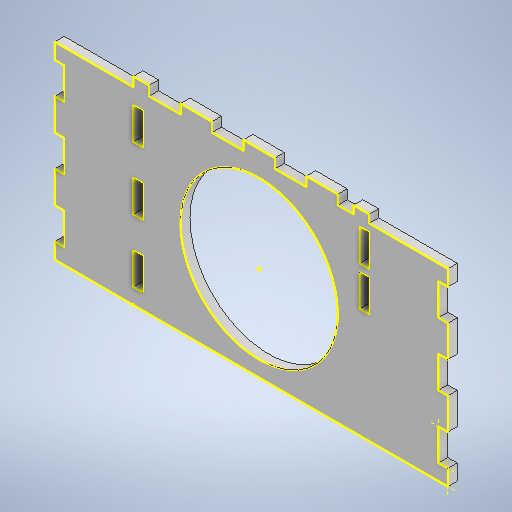
# Autodesk Inventor part: Archimedes Screw Border1
Saved by Autodesk Inventor 2025.3 (Build 293356000, 356)
## iProperties
Created: 2026-03-14
Part Number: Archimedes Screw Border1
Material: Generic
Document SubType Name: Modeling
Designer: ziada
Density: 1 g/cm^3
Appearance: Default
Author: ziada
Autodesk Inventor part; units mm, degrees
ref_plane "YZ Plane" through (0, 0, 0) normal (1, 0, 0) x (0, 1, 0)
ref_plane "XZ Plane" through (0, 0, 0) normal (0, 1, 0) x (-1, 0, 0)
ref_plane "XY Plane" through (0, 0, 0) normal (0, 0, 1) x (1, 0, 0)
sketch "Sketch1" plane through (0, 0, 0) normal (0, 0, 1) x (1, 0, 0)
  line L0 (0, 0) -> (0, 120)
  circle A0 centre (80, 60) radius 50
  line L1 (0, 0) -> (150, 0)
  line L2 (150, 120) -> (0, 120)
  line L3 (0, 120) -> (0, 110)
  line L4 (0, 110) -> (6, 110)
  line L5 (6, 110) -> (6, 90)
  line L6 (6, 90) -> (0, 90)
  line L7 (0, 90) -> (0, 70)
  line L8 (0, 70) -> (6, 70)
  line L9 (6, 70) -> (6, 50)
  line L10 (6, 50) -> (0, 50)
  line L11 (0, 50) -> (0, 30)
  line L12 (0, 30) -> (6, 30)
  line L13 (6, 30) -> (6, 10)
  line L14 (6, 10) -> (0, 10)
  line L15 (0, 120) -> (-50, 120)
  line L16 (-50, 120) -> (-50, 110)
  line L17 (-50, 110) -> (-44, 110)
  line L18 (-44, 110) -> (-44, 90)
  line L19 (-44, 90) -> (-50, 90)
  line L20 (-50, 90) -> (-50, 70)
  line L21 (-50, 70) -> (-44, 70)
  line L22 (-44, 70) -> (-44, 50)
  line L23 (-44, 50) -> (-50, 50)
  line L24 (-50, 50) -> (-50, 30)
  line L25 (-50, 30) -> (-44, 30)
  line L26 (-44, 30) -> (-44, 10)
  line L27 (-44, 10) -> (-50, 10)
  line L28 (-50, 10) -> (-50, 0)
  line L29 (-50, 0) -> (0, 0)
  line L30 (150, 115) -> (144, 115)
  line L31 (144, 115) -> (144, 95)
  line L32 (150, 120) -> (200, 120)
  line L33 (200, 120) -> (200, 110)
  line L34 (200, 110) -> (194, 110)
  line L35 (194, 110) -> (194, 90)
  line L36 (194, 90) -> (200, 90)
  line L37 (200, 90) -> (200, 70)
  line L38 (200, 70) -> (194, 70)
  line L39 (194, 70) -> (194, 50)
  line L40 (194, 50) -> (200, 50)
  line L41 (200, 50) -> (200, 30)
  line L42 (200, 30) -> (194, 30)
  line L43 (194, 30) -> (194, 10)
  line L44 (194, 10) -> (200, 10)
  line L45 (200, 10) -> (200, 0)
  line L46 (200, 0) -> (150, 0)
  line L47 (150, 120) -> (150, 0)
  line L48 (144, 95) -> (150, 95)
  line L49 (150, 95) -> (150, 90)
  line L50 (150, 90) -> (144, 90)
  line L51 (144, 90) -> (144, 70)
  line L52 (144, 70) -> (150, 70)
  line L53 (0, 120) -> (0, 126)
  line L54 (150, 125) -> (150, 120)
  line L55 (0, 126) -> (10, 126)
  line L56 (10, 126) -> (10, 120)
  line L57 (10, 120) -> (30, 120)
  line L58 (30, 120) -> (30, 126)
  line L59 (30, 126) -> (50, 126)
  line L60 (50, 126) -> (50, 120)
  line L61 (50, 120) -> (70, 120)
  line L62 (70, 120) -> (70, 126)
  line L63 (70, 126) -> (90, 126)
  line L64 (90, 126) -> (90, 120)
  line L65 (90, 120) -> (110, 120)
  line L66 (110, 120) -> (110, 126)
  line L67 (110, 126) -> (130, 126)
  line L68 (130, 126) -> (130, 120)
  line L69 (130, 120) -> (140, 120)
  line L70 (140, 120) -> (140, 125)
  line L71 (140, 125) -> (150, 125)
  dimension "d12" = 100
  dimension "d13" = 120
  dimension "d14" = 150
  dimension "d17" = 80
  dimension "d18" = 60
  dimension "d19" = 10
  dimension "d20" = 6
  dimension "d21" = 20
  dimension "d22" = 20
  dimension "d24" = 20
  dimension "d25" = 20
  dimension "d26" = 20
  dimension "d38" = 50
  dimension "d39" = 10
  dimension "d40" = 6
  dimension "d41" = 5
  dimension "d42" = 6
  dimension "d43" = 50
  dimension "d44" = 6
  dimension "d45" = 5
  dimension "d46" = 20
  dimension "d47" = 20
  dimension "d48" = 6
  dimension "d51" = 10
  dimension "d52" = 20
  dimension "d53" = 20
  dimension "d54" = 20
  dimension "d55" = 20
  dimension "d56" = 20
  dimension "d57" = 20
  dimension "d58" = 10
  constraints: 142 end point, 39 point on line, 31 perpendicular, 8 vertical, 6 horizontal, 1 centre point, 1 parallel, 11 other
  measures "d12" diameter of A0
  measures "d13" distance of L0.start L0.end
  measures "d14" distance of L32.start L0.end
  measures "d17" distance from line of L0 A0.centre
  measures "d19" distance of L0.end L3.end
  measures "d20" distance of L3.end L4.end
  measures "d21" distance of L4.end L5.end
  measures "d22" distance of L6.end L7.end
  measures "d24" distance of L8.end L9.end
  measures "d25" distance of L10.end L11.end
  measures "d26" distance of L12.end L13.end
  measures "d38" distance of L0.end L15.end
  measures "d39" distance of L15.end L16.end
  measures "d40" distance of L16.end L17.end
  measures "d41" distance of L32.start L30.start
  measures "d42" distance of L30.start L30.end
  measures "d43" distance of L32.start L32.end
  measures "d44" distance of L33.end L34.end
  measures "d45" distance between parallel lines of L50 L48
  measures "d46" distance of L50.end L51.end
  measures "d47" distance of L30.end L31.end
  measures "d48" distance of L0.end L53.end
  measures "d51" distance of L53.end L55.end
  measures "d52" distance of L56.end L57.end
  measures "d53" distance of L58.end L59.end
  measures "d54" distance of L60.end L61.end
  measures "d55" distance of L62.end L63.end
  measures "d56" distance of L64.end L65.end
  measures "d57" distance of L66.end L67.end
  measures "d58" distance of L68.end L69.end
extrude "Extrusion1" add sketch "Sketch1" against normal blind 6 contours L29 L28 L27 L26 L25 L24 L23 L22 L21 L20 L19 L18 L17 L16 L15 L0 | L0 L14 L13 L12 L10 L9 L8 L6 L5 L4 L2 L47 L30 L31 L48 L50 L51 L52 L1 | L47 L32 L33 L34 L35 L36 L37 L38 L39 L40 L41 L42 L43 L44 L45 L46
extrude "Extrusion3" add sketch "Sketch1" against normal blind 6 contours L2 L70 L71 L54 | L53 L55 L56 L2 | L2 L66 L67 L68 | L58 L59 L60 L2 | L2 L62 L63 L64
sketch "Sketch3" plane through (0, 0, 0) normal (0, 0, 1) x (1, 0, 0)
  line L0 (200, 30) -> (200, 50) projected
  line L1 (194, 30) -> (200, 30) projected
  line L2 (200, 50) -> (200, 30) projected
  line L3 (200, 30) -> (194, 30) projected
  line L4 (194, 10) -> (194, 30) projected
  line L5 (194, 30) -> (194, 10) projected
  line L6 (200, 10) -> (194, 10) projected
  line L7 (194, 10) -> (200, 10) projected
  line L8 (200, 0) -> (200, 10) projected
  circle A0 centre (80, 60) radius 50 projected
  circle A1 centre (80, 60) radius 50 projected
  circle A2 centre (80, 60) radius 50 projected
  circle A3 centre (80, 60) radius 50 projected
  line L9 (0, 30) -> (6, 30) projected
  line L10 (6, 30) -> (6, 10) projected
  line L11 (6, 10) -> (0, 10) projected
  line L12 (0, 10) -> (0, 30) projected
  circle A4 centre (80, 60) radius 50 projected
  line L13 (150, 90) -> (150, 70) projected
  line L14 (150, 70) -> (144, 70) projected
  line L15 (144, 70) -> (144, 90) projected
  line L16 (144, 90) -> (150, 90) projected
  line L17 (150, 115) -> (150, 95) projected
  line L18 (150, 95) -> (144, 95) projected
  line L19 (144, 95) -> (144, 115) projected
  line L20 (144, 115) -> (150, 115) projected
  line L21 (0, 70) -> (6, 70) projected
  line L22 (6, 70) -> (6, 50) projected
  line L23 (6, 50) -> (0, 50) projected
  line L24 (0, 50) -> (0, 70) projected
  line L25 (0, 110) -> (6, 110) projected
  line L26 (6, 110) -> (6, 90) projected
  line L27 (6, 90) -> (0, 90) projected
  line L28 (0, 90) -> (0, 110) projected
  line L29 (200, 120) -> (150, 120) projected
  line L30 (150, 120) -> (150, 125) projected
  line L31 (150, 125) -> (140, 125) projected
  line L32 (140, 125) -> (140, 120) projected
  line L33 (140, 120) -> (130, 120) projected
  line L34 (130, 120) -> (130, 126) projected
  line L35 (130, 126) -> (110, 126) projected
  line L36 (110, 126) -> (110, 120) projected
  line L37 (110, 120) -> (90, 120) projected
  line L38 (90, 120) -> (90, 126) projected
  line L39 (90, 126) -> (70, 126) projected
  line L40 (70, 126) -> (70, 120) projected
  line L41 (70, 120) -> (50, 120) projected
  line L42 (50, 120) -> (50, 126) projected
  line L43 (50, 126) -> (30, 126) projected
  line L44 (30, 126) -> (30, 120) projected
  line L45 (30, 120) -> (10, 120) projected
  line L46 (10, 120) -> (10, 126) projected
  line L47 (10, 126) -> (0, 126) projected
  line L48 (0, 126) -> (0, 120) projected
  line L49 (0, 120) -> (-50, 120) projected
  line L50 (-50, 120) -> (-50, 110) projected
  line L51 (-50, 110) -> (-44, 110) projected
  line L52 (-44, 110) -> (-44, 90) projected
  line L53 (-44, 90) -> (-50, 90) projected
  line L54 (-50, 90) -> (-50, 70) projected
  line L55 (-50, 70) -> (-44, 70) projected
  line L56 (-44, 70) -> (-44, 50) projected
  line L57 (-44, 50) -> (-50, 50) projected
  line L58 (-50, 50) -> (-50, 30) projected
  line L59 (-50, 30) -> (-44, 30) projected
  line L60 (-44, 30) -> (-44, 10) projected
  line L61 (-44, 10) -> (-50, 10) projected
  line L62 (-50, 10) -> (-50, 0) projected
  line L63 (-50, 0) -> (200, 0) projected
  line L64 (200, 0) -> (200, 10) projected
  line L65 (200, 10) -> (194, 10) projected
  line L66 (194, 10) -> (194, 30) projected
  line L67 (194, 30) -> (200, 30) projected
  line L68 (200, 30) -> (200, 50) projected
  line L69 (200, 50) -> (194, 50) projected
  line L70 (194, 50) -> (194, 70) projected
  line L71 (194, 70) -> (200, 70) projected
  line L72 (200, 70) -> (200, 90) projected
  line L73 (200, 90) -> (194, 90) projected
  line L74 (194, 90) -> (194, 110) projected
  line L75 (194, 110) -> (200, 110) projected
  line L76 (200, 110) -> (200, 120) projected
  line L77 (6, 30) -> (0, 30) projected
  line L78 (0, 30) -> (0, 10) projected
  line L79 (0, 10) -> (6, 10) projected
  line L80 (6, 10) -> (6, 30) projected
  circle A5 centre (80, 60) radius 50 projected
  line L81 (150, 70) -> (150, 90) projected
  line L82 (150, 90) -> (144, 90) projected
  line L83 (144, 90) -> (144, 70) projected
  line L84 (144, 70) -> (150, 70) projected
  line L85 (150, 95) -> (150, 115) projected
  line L86 (150, 115) -> (144, 115) projected
  line L87 (144, 115) -> (144, 95) projected
  line L88 (144, 95) -> (150, 95) projected
  line L89 (6, 70) -> (0, 70) projected
  line L90 (0, 70) -> (0, 50) projected
  line L91 (0, 50) -> (6, 50) projected
  line L92 (6, 50) -> (6, 70) projected
  line L93 (6, 110) -> (0, 110) projected
  line L94 (0, 110) -> (0, 90) projected
  line L95 (0, 90) -> (6, 90) projected
  line L96 (6, 90) -> (6, 110) projected
  line L97 (-50, 120) -> (0, 120) projected
  line L98 (0, 120) -> (0, 126) projected
  line L99 (0, 126) -> (10, 126) projected
  line L100 (10, 126) -> (10, 120) projected
  line L101 (10, 120) -> (30, 120) projected
  line L102 (30, 120) -> (30, 126) projected
  line L103 (30, 126) -> (50, 126) projected
  line L104 (50, 126) -> (50, 120) projected
  line L105 (50, 120) -> (70, 120) projected
  line L106 (70, 120) -> (70, 126) projected
  line L107 (70, 126) -> (90, 126) projected
  line L108 (90, 126) -> (90, 120) projected
  line L109 (90, 120) -> (110, 120) projected
  line L110 (110, 120) -> (110, 126) projected
  line L111 (110, 126) -> (130, 126) projected
  line L112 (130, 126) -> (130, 120) projected
  line L113 (130, 120) -> (140, 120) projected
  line L114 (140, 120) -> (140, 125) projected
  line L115 (140, 125) -> (150, 125) projected
  line L116 (150, 125) -> (150, 120) projected
  line L117 (150, 120) -> (200, 120) projected
  line L118 (200, 120) -> (200, 110) projected
  line L119 (200, 110) -> (194, 110) projected
  line L120 (194, 110) -> (194, 90) projected
  line L121 (194, 90) -> (200, 90) projected
  line L122 (200, 90) -> (200, 70) projected
  line L123 (200, 70) -> (194, 70) projected
  line L124 (194, 70) -> (194, 50) projected
  line L125 (194, 50) -> (200, 50) projected
  line L126 (200, 50) -> (200, 30) projected
  line L127 (200, 30) -> (194, 30) projected
  line L128 (194, 30) -> (194, 10) projected
  line L129 (194, 10) -> (200, 10) projected
  line L130 (200, 10) -> (200, 0) projected
  line L131 (200, 0) -> (-50, 0) projected
  line L132 (-50, 0) -> (-50, 10) projected
  line L133 (-50, 10) -> (-44, 10) projected
  line L134 (-44, 10) -> (-44, 30) projected
  line L135 (-44, 30) -> (-50, 30) projected
  line L136 (-50, 30) -> (-50, 50) projected
  line L137 (-50, 50) -> (-44, 50) projected
  line L138 (-44, 50) -> (-44, 70) projected
  line L139 (-44, 70) -> (-50, 70) projected
  line L140 (-50, 70) -> (-50, 90) projected
  line L141 (-50, 90) -> (-44, 90) projected
  line L142 (-44, 90) -> (-44, 110) projected
  line L143 (-44, 110) -> (-50, 110) projected
  line L144 (-50, 110) -> (-50, 120) projected
  line L145 (-50, 0) -> (200, 0) projected
  line L146 (200, 0) -> (-50, 0) projected
  line L147 (-50, 0) -> (200, 0) projected
  line L148 (200, 0) -> (-50, 0) projected
  line L149 (200, 10) -> (200, 0) projected
  line L150 (200, 90) -> (194, 90) projected
  line L151 (194, 90) -> (200, 90) projected
  line L152 (194, 50) -> (200, 50) projected
  line L153 (200, 110) -> (194, 110) projected
  line L154 (194, 110) -> (200, 110) projected
  line L155 (200, 120) -> (200, 110) projected
  line L156 (200, 110) -> (200, 120) projected
  line L157 (200, 50) -> (194, 50) projected
  line L158 (194, 110) -> (194, 90) projected
  line L159 (194, 70) -> (194, 50) projected
  line L160 (194, 90) -> (194, 110) projected
  line L161 (194, 50) -> (194, 70) projected
  line L162 (200, 90) -> (200, 70) projected
  line L163 (200, 70) -> (200, 90) projected
  line L164 (194, 70) -> (200, 70) projected
  line L165 (6, 50) -> (0, 50) projected
  line L166 (6, 50) -> (6, 70) projected
  line L167 (6, 70) -> (6, 50) projected
  line L168 (0, 70) -> (0, 50) projected
  line L169 (-44, 70) -> (-44, 50) projected
  line L170 (0, 50) -> (0, 70) projected
  line L171 (200, 70) -> (194, 70) projected
  line L172 (70, 120) -> (70, 126) projected
  line L173 (70, 126) -> (70, 120) projected
  line L174 (70, 126) -> (90, 126) projected
  line L175 (90, 126) -> (70, 126) projected
  line L176 (90, 126) -> (90, 120) projected
  line L177 (90, 120) -> (90, 126) projected
  line L178 (110, 126) -> (110, 120) projected
  line L179 (110, 120) -> (110, 126) projected
  line L180 (110, 120) -> (90, 120) projected
  line L181 (90, 120) -> (110, 120) projected
  line L182 (90, 120) -> (90, 126) projected
  line L183 (90, 126) -> (90, 120) projected
  line L184 (90, 126) -> (70, 126) projected
  line L185 (70, 126) -> (90, 126) projected
  line L186 (90, 120) -> (110, 120) projected
  line L187 (110, 120) -> (90, 120) projected
  line L188 (130, 120) -> (140, 120) projected
  line L189 (140, 120) -> (130, 120) projected
  line L190 (110, 120) -> (110, 126) projected
  line L191 (110, 126) -> (110, 120) projected
  line L192 (110, 126) -> (130, 126) projected
  line L193 (130, 126) -> (110, 126) projected
  line L194 (130, 126) -> (130, 120) projected
  line L195 (130, 120) -> (130, 126) projected
  line L196 (140, 125) -> (150, 125) projected
  line L197 (150, 125) -> (140, 125) projected
  line L198 (150, 125) -> (150, 120) projected
  line L199 (150, 120) -> (150, 125) projected
  line L200 (150, 120) -> (150, 125) projected
  line L201 (150, 125) -> (150, 120) projected
  line L202 (150, 125) -> (140, 125) projected
  line L203 (140, 125) -> (150, 125) projected
  line L204 (140, 120) -> (140, 125) projected
  line L205 (140, 125) -> (140, 120) projected
  line L206 (140, 125) -> (140, 120) projected
  line L207 (140, 120) -> (140, 125) projected
  line L208 (130, 120) -> (140, 120) projected
  line L209 (140, 120) -> (130, 120) projected
  line L210 (130, 120) -> (130, 126) projected
  line L211 (130, 126) -> (130, 120) projected
  line L212 (130, 126) -> (110, 126) projected
  line L213 (110, 126) -> (130, 126) projected
  line L214 (150, 70) -> (150, 90) projected
  line L215 (150, 90) -> (150, 70) projected
  line L216 (150, 90) -> (144, 90) projected
  line L217 (144, 90) -> (150, 90) projected
  line L218 (144, 90) -> (144, 70) projected
  line L219 (144, 70) -> (144, 90) projected
  line L220 (144, 70) -> (150, 70) projected
  line L221 (150, 70) -> (144, 70) projected
  line L222 (144, 70) -> (144, 90) projected
  line L223 (144, 90) -> (144, 70) projected
  line L224 (144, 90) -> (150, 90) projected
  line L225 (150, 90) -> (144, 90) projected
  line L226 (150, 95) -> (144, 95) projected
  line L227 (144, 95) -> (150, 95) projected
  line L228 (150, 115) -> (150, 95) projected
  line L229 (150, 95) -> (150, 115) projected
  line L230 (144, 95) -> (144, 115) projected
  line L231 (144, 115) -> (144, 95) projected
  line L232 (144, 115) -> (150, 115) projected
  line L233 (150, 115) -> (144, 115) projected
  line L234 (150, 70) -> (144, 70) projected
  line L235 (144, 70) -> (150, 70) projected
  line L236 (150, 90) -> (150, 70) projected
  line L237 (150, 70) -> (150, 90) projected
  line L238 (150, 120) -> (200, 120) projected
  line L239 (200, 120) -> (150, 120) projected
  line L240 (200, 120) -> (150, 120) projected
  line L241 (150, 120) -> (200, 120) projected
  line L242 (194, 90) -> (194, 110) projected
  line L243 (194, 110) -> (194, 90) projected
  line L244 (194, 110) -> (200, 110) projected
  line L245 (200, 110) -> (194, 110) projected
  line L246 (200, 90) -> (194, 90) projected
  line L247 (194, 90) -> (200, 90) projected
  line L248 (200, 70) -> (200, 90) projected
  line L249 (200, 90) -> (200, 70) projected
  line L250 (200, 50) -> (194, 50) projected
  line L251 (194, 50) -> (200, 50) projected
  line L252 (200, 30) -> (200, 50) projected
  line L253 (200, 50) -> (200, 30) projected
  line L254 (194, 30) -> (200, 30) projected
  line L255 (200, 30) -> (194, 30) projected
  line L256 (194, 10) -> (194, 30) projected
  line L257 (194, 30) -> (194, 10) projected
  line L258 (200, 0) -> (200, 10) projected
  line L259 (200, 10) -> (200, 0) projected
  line L260 (200, 10) -> (194, 10) projected
  line L261 (194, 10) -> (200, 10) projected
  line L262 (194, 50) -> (194, 70) projected
  line L263 (194, 70) -> (194, 50) projected
  line L264 (194, 70) -> (200, 70) projected
  line L265 (200, 70) -> (194, 70) projected
  line L266 (200, 110) -> (200, 120) projected
  line L267 (200, 120) -> (200, 110) projected
  line L268 (150, 95) -> (150, 115) projected
  line L269 (150, 115) -> (150, 95) projected
  line L270 (150, 115) -> (144, 115) projected
  line L271 (144, 115) -> (150, 115) projected
  line L272 (144, 115) -> (144, 95) projected
  line L273 (144, 95) -> (144, 115) projected
  line L274 (144, 95) -> (150, 95) projected
  line L275 (150, 95) -> (144, 95) projected
  line L276 (30, 120) -> (10, 120) projected
  line L277 (10, 120) -> (30, 120) projected
  line L278 (30, 126) -> (30, 120) projected
  line L279 (30, 120) -> (30, 126) projected
  line L280 (50, 126) -> (30, 126) projected
  line L281 (30, 126) -> (50, 126) projected
  line L282 (50, 120) -> (70, 120) projected
  line L283 (70, 120) -> (50, 120) projected
  line L284 (70, 126) -> (70, 120) projected
  line L285 (70, 120) -> (70, 126) projected
  line L286 (50, 120) -> (50, 126) projected
  line L287 (50, 126) -> (50, 120) projected
  line L288 (50, 120) -> (70, 120) projected
  line L289 (70, 120) -> (50, 120) projected
  line L290 (6, 90) -> (6, 110) projected
  line L291 (6, 10) -> (6, 30) projected
  line L292 (50, 126) -> (50, 120) projected
  line L293 (30, 126) -> (30, 120) projected
  line L294 (30, 126) -> (50, 126) projected
  line L295 (50, 126) -> (30, 126) projected
  line L296 (50, 120) -> (50, 126) projected
  line L297 (0, 10) -> (0, 30) projected
  line L298 (0, 110) -> (0, 90) projected
  line L299 (0, 90) -> (0, 110) projected
  line L300 (6, 90) -> (0, 90) projected
  line L301 (6, 110) -> (6, 90) projected
  line L302 (0, 90) -> (6, 90) projected
  line L303 (0, 50) -> (6, 50) projected
  line L304 (0, 110) -> (6, 110) projected
  line L305 (6, 110) -> (0, 110) projected
  line L306 (10, 120) -> (10, 126) projected
  line L307 (0, 126) -> (0, 120) projected
  line L308 (10, 126) -> (0, 126) projected
  line L309 (0, 120) -> (0, 126) projected
  line L310 (0, 126) -> (10, 126) projected
  line L311 (10, 126) -> (10, 120) projected
  line L312 (10, 120) -> (30, 120) projected
  line L313 (30, 120) -> (10, 120) projected
  line L314 (0, 120) -> (-50, 120) projected
  line L315 (-50, 120) -> (0, 120) projected
  line L316 (30, 120) -> (30, 126) projected
  line L317 (-44, 50) -> (-44, 70) projected
  line L318 (-44, 70) -> (-50, 70) projected
  line L319 (-50, 70) -> (-44, 70) projected
  line L320 (-50, 70) -> (-50, 90) projected
  line L321 (-50, 90) -> (-50, 70) projected
  line L322 (-50, 90) -> (-44, 90) projected
  line L323 (-44, 90) -> (-50, 90) projected
  line L324 (-44, 90) -> (-44, 110) projected
  line L325 (6, 70) -> (0, 70) projected
  line L326 (0, 70) -> (6, 70) projected
  line L327 (-44, 110) -> (-44, 90) projected
  line L328 (-50, 110) -> (-44, 110) projected
  line L329 (-44, 110) -> (-50, 110) projected
  line L330 (-50, 120) -> (-50, 110) projected
  line L331 (-50, 110) -> (-50, 120) projected
  line L332 (-50, 10) -> (-50, 0) projected
  line L333 (-50, 0) -> (-50, 10) projected
  line L334 (-44, 10) -> (-50, 10) projected
  line L335 (-50, 10) -> (-44, 10) projected
  line L336 (10, 120) -> (10, 126) projected
  line L337 (10, 126) -> (10, 120) projected
  line L338 (10, 126) -> (0, 126) projected
  line L339 (0, 126) -> (10, 126) projected
  line L340 (0, 126) -> (0, 120) projected
  line L341 (0, 120) -> (0, 126) projected
  line L342 (0, 110) -> (6, 110) projected
  line L343 (6, 110) -> (0, 110) projected
  line L344 (6, 110) -> (6, 90) projected
  line L345 (6, 90) -> (6, 110) projected
  line L346 (0, 90) -> (0, 110) projected
  line L347 (0, 110) -> (0, 90) projected
  line L348 (6, 90) -> (0, 90) projected
  line L349 (0, 90) -> (6, 90) projected
  line L350 (0, 70) -> (6, 70) projected
  line L351 (6, 70) -> (0, 70) projected
  line L352 (6, 70) -> (6, 50) projected
  line L353 (6, 50) -> (6, 70) projected
  line L354 (0, 50) -> (0, 70) projected
  line L355 (0, 70) -> (0, 50) projected
  line L356 (6, 50) -> (0, 50) projected
  line L357 (0, 50) -> (6, 50) projected
  line L358 (-50, 120) -> (0, 120) projected
  line L359 (0, 120) -> (-50, 120) projected
  line L360 (-50, 120) -> (-50, 110) projected
  line L361 (-50, 110) -> (-50, 120) projected
  line L362 (-44, 110) -> (-44, 90) projected
  line L363 (-44, 90) -> (-44, 110) projected
  line L364 (-50, 110) -> (-44, 110) projected
  line L365 (-44, 110) -> (-50, 110) projected
  line L366 (0, 30) -> (6, 30) projected
  line L367 (6, 30) -> (0, 30) projected
  line L368 (-44, 90) -> (-50, 90) projected
  line L369 (-50, 90) -> (-44, 90) projected
  line L370 (-50, 90) -> (-50, 70) projected
  line L371 (-50, 70) -> (-50, 90) projected
  line L372 (6, 30) -> (6, 10) projected
  line L373 (6, 10) -> (6, 30) projected
  line L374 (6, 10) -> (0, 10) projected
  line L375 (0, 10) -> (6, 10) projected
  line L376 (0, 10) -> (0, 30) projected
  line L377 (0, 30) -> (0, 10) projected
  line L378 (-50, 70) -> (-44, 70) projected
  line L379 (-44, 70) -> (-50, 70) projected
  line L380 (-44, 70) -> (-44, 50) projected
  line L381 (-44, 50) -> (-44, 70) projected
  line L382 (-44, 50) -> (-50, 50) projected
  line L383 (-50, 50) -> (-44, 50) projected
  line L384 (-50, 50) -> (-50, 30) projected
  line L385 (-50, 30) -> (-50, 50) projected
  line L386 (-44, 30) -> (-44, 10) projected
  line L387 (-44, 10) -> (-44, 30) projected
  line L388 (-50, 30) -> (-44, 30) projected
  line L389 (-44, 30) -> (-50, 30) projected
  line L390 (-50, 50) -> (-50, 30) projected
  line L391 (-44, 10) -> (-44, 30) projected
  line L392 (-44, 50) -> (-50, 50) projected
  line L393 (-50, 50) -> (-44, 50) projected
  line L394 (-50, 30) -> (-50, 50) projected
  line L395 (-44, 30) -> (-50, 30) projected
  line L396 (-50, 30) -> (-44, 30) projected
  line L397 (-44, 30) -> (-44, 10) projected
  line L398 (-50, 10) -> (-44, 10) projected
  line L399 (-50, 0) -> (-50, 10) projected
  line L400 (0, 30) -> (0, 10) projected
  line L401 (-44, 10) -> (-50, 10) projected
  line L402 (6, 30) -> (0, 30) projected
  line L403 (0, 10) -> (6, 10) projected
  line L404 (0, 30) -> (6, 30) projected
  line L405 (6, 30) -> (6, 10) projected
  line L406 (6, 10) -> (0, 10) projected
  line L407 (-50, 10) -> (-50, 0) projected
  point P0 (0, 0)
  constraints: 42 other
body "Solid1"
